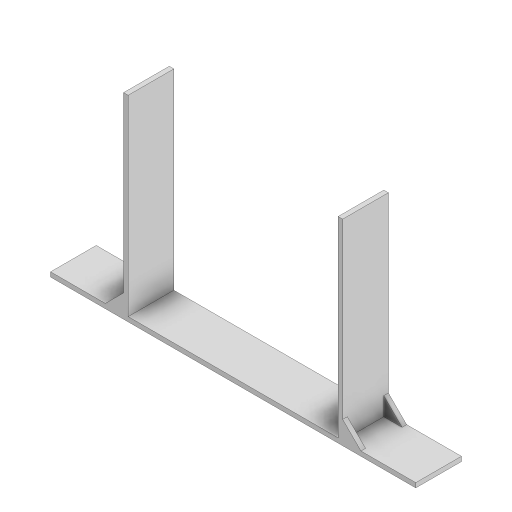
# Autodesk Inventor part: SOPORTE DE GUIA
Saved by Autodesk Inventor 2024 (Build 280153000, 153)
## iProperties
Created: 2024-05-26
Part Number: SOPORTE DE GUIA
Material: Generic
Document SubType Name: Modeling
Designer: Jhuliams
Density: 1 g/cm^3
Appearance: Default
Author: Jhuliams
Autodesk Inventor part; units mm, degrees
ref_plane "YZ Plane" through (0, 0, 0) normal (1, 0, 0) x (0, 1, 0)
ref_plane "XZ Plane" through (0, 0, 0) normal (0, 1, 0) x (-1, 0, 0)
ref_plane "XY Plane" through (0, 0, 0) normal (0, 0, 1) x (1, 0, 0)
sketch "Sketch1" plane through (0, 0, 0) normal (0, 0, 1) x (1, 0, 0)
  line L0 (-60, 52.5) -> (60, 52.5)
  line L1 (60, 52.5) -> (60, -52.5)
  line L2 (60, -52.5) -> (-60, -52.5)
  line L3 (-60, -52.5) -> (-60, 52.5)
  line L4 (-60, 52.5) -> (60, -52.5) construction
  line L5 (60, 52.5) -> (-60, -52.5) construction
  circle A0 centre (0, 0) radius 52.5
  line L6 (-52.5, 0) -> (-60, 0)
  line L7 (52.5, 0) -> (60, 0)
  line L8 (-100, -55) -> (100, -55)
  line L9 (100, -55) -> (100, -50)
  line L10 (100, -50) -> (-100, -50)
  line L11 (-100, -50) -> (-100, -55)
  line L12 (-100, -55) -> (100, -50) construction
  line L13 (100, -55) -> (-100, -50) construction
  line L14 (-57.5, 52.5) -> (57.5, 52.5)
  line L15 (57.5, 52.5) -> (57.5, -52.5)
  line L16 (57.5, -52.5) -> (-57.5, -52.5)
  line L17 (-57.5, -52.5) -> (-57.5, 52.5)
  line L18 (-57.5, 52.5) -> (57.5, -52.5) construction
  line L19 (57.5, 52.5) -> (-57.5, -52.5) construction
  line L20 (-100, -52.5) -> (100, -52.5)
  point P0 (0, -52.5)
  point P1 (-60, -50)
  point P2 (60, -50)
  point P3 (60, -52.5)
  point P4 (57.5, 52.5)
  point P5 (57.5, -52.5)
  point P6 (-57.5, 52.5)
  point P7 (-60, -52.5)
  dimension "d0" = 120
  dimension "d1" = 105
  dimension "d2" = 105
  dimension "d5" = 200
  dimension "d6" = 5
  dimension "d30" = 115
  dimension "d31" = 105
  constraints: 42 end point, 11 midpoint, 6 parallel, 3 horizontal, 3 perpendicular, 2 point on circle, 1 centre point, 1 coincident, 1 point on line
  measures "d0" distance of L1.end L2.end
  measures "d1" distance of L0.end L1.end
  measures "d2" diameter of A0
  measures "d5" distance of L10.end L9.end
  measures "d6" distance of L9.end L8.end
  measures "d30" distance of L15.end L16.end
  measures "d31" distance of L14.end L15.end
extrude "Extrusion1" add sketch "Sketch1" along normal mid plane 25 contours L0 L17 L6 L3 | L6 L17 L10 L3 | L10 L17 L2 L3 | L0 L1 L7 L15 | L2 L20 L9 L8 L11 | L7 L1 L10 L15 | L10 L1 L2 L15
sketch "Sketch6" plane through (0, 0, 12.5) normal (0, 0, 1) x (1, 0, 0)
  line L0 (-60, -52.5) -> (-60, -42.5)
  line L1 (-60, 52.5) -> (-60, -52.5) projected
  line L2 (-60, -52.5) -> (-70, -52.5)
  line L3 (-60, -52.5) -> (-100, -52.5) projected
  line L4 (-70, -52.5) -> (-60, -42.5)
  line L5 (0, -52.5) -> (0, -39.6875)
  line L6 (60, -52.5) -> (60, -42.5)
  line L7 (60, -52.5) -> (70, -52.5)
  line L8 (70, -52.5) -> (60, -42.5)
  point P0 (0, 0)
  dimension "d32" = 10
  dimension "d33" = 10
  constraints: 14 end point, 3 symmetric about line, 2 point on line, 1 vertical
  measures "d32" distance of L0.start L0.end
  measures "d33" distance of L0.start L2.end
extrude "Extrusion5" add sketch "Sketch6" against normal blind 2.5
mirror "Mirror1" about plane through (0, 0, 0) normal (0, 0, 1) of "Extrusion5"
body "Solid1"
